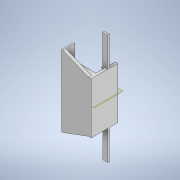
# Autodesk Inventor part: gira
Saved by Autodesk Inventor 2020 (Build 240168000, 168)
## iProperties
Created: 2022-10-31
Part Number: gira
Material: Generic
Document SubType Name: Modeling
Designer: super
Density: 1 g/cm^3
Appearance: Default
Author: super
Autodesk Inventor part; units mm, degrees
ref_plane "YZ Plane" through (0, 0, 0) normal (1, 0, 0) x (0, 1, 0)
ref_plane "XZ Plane" through (0, 0, 0) normal (0, 1, 0) x (-1, 0, 0)
ref_plane "XY Plane" through (0, 0, 0) normal (0, 0, 1) x (1, 0, 0)
ref_plane "Work Plane1" through (-84.5679, -177.7614, 10.4079) normal (0.999999, 0.0014131, 0) x (0.0014131, -0.999999, 0)
sketch "Sketch1" plane through (-84.5679, -177.7614, 10.4079) normal (0.999999, 0.0014131, 0) x (0.0014131, -0.999999, 0)
  line L0 (9.6295, -13.989) -> (-230.3705, -13.989)
  line L1 (-230.3705, -13.989) -> (-230.3705, 16.011)
  line L2 (-230.3705, 16.011) -> (9.6295, 16.011)
  line L3 (9.6295, 16.011) -> (9.6295, -13.989)
  point P0 (-177.6417, 10.4079)
  dimension "d40" = 240
  dimension "d41" = 30
  constraints: 8 end point, 2 parallel, 1 horizontal, 1 perpendicular
  measures "d40" distance of L0.start L0.end
  measures "d41" distance of L2.end L0.start
extrude "Extrusion1" add sketch "Sketch1" along normal blind 5
ref_plane "Work Plane2" through (-84.7238, -67.391, 24.3968) normal (-0.0014131, 0.999999, 0) x (0.999999, 0.0014131, 0)
sketch "Sketch3" plane through (-84.5543, -187.3909, 24.3968) normal (0, 0, 1) x (0.999999, 0.0014131, 0)
  line L0 (0, 0) -> (5, 0)
  line L1 (5, 0) -> (91.2544, 31.8306)
  line L2 (91.2544, 31.8306) -> (100.3623, 31.8306)
  line L3 (100.3623, 31.8306) -> (100.3623, 204.35)
  line L4 (100.3623, 204.35) -> (91.2544, 204.35)
  line L5 (5, 0) -> (5, 240) projected
  line L6 (91.2544, 204.35) -> (5, 240)
  line L7 (0, 0) -> (0, 240) projected
  line L8 (5, 240) -> (0, 240)
  line L9 (0, 240) -> (0, 0)
  point P0 (84.819, 187.2712)
  dimension "d42" = 172.5194
  dimension "d43" = 35.65
  constraints: 16 end point, 3 perpendicular, 2 parallel, 1 horizontal
  measures "d42" distance of L2.end L3.end
  measures "d43" vertical distance of L4.end L5.end
extrude "Extrusion2" add sketch "Sketch3" along normal blind 10
sketch "Sketch4" plane through (-84.5543, -187.3909, 24.3968) normal (0, 0, -1) x (-0.999999, -0.0014131, 0)
  line L0 (-100.3623, 204.35) -> (-91.2544, 204.35) projected
  line L1 (-91.2544, 31.8306) -> (-100.3623, 31.8306) projected
  line L2 (-100.3623, 204.35) -> (-91.2544, 204.35)
  line L3 (-91.2544, 204.35) -> (-91.2544, 31.8306)
  line L4 (-91.2544, 31.8306) -> (-100.3623, 31.8306)
  line L5 (-100.3623, 31.8306) -> (-100.3623, 204.35)
  point P0 (-84.819, 187.2712)
  point P1 (-100.3623, 31.8306)
  constraints: 8 end point, 2 parallel, 1 horizontal, 1 perpendicular
extrude "Extrusion3" add sketch "Sketch4" along normal blind 80
sketch "Sketch6" plane through (15.7629, -155.4186, -55.6032) normal (0.0014131, -0.999999, 0) x (0.999999, 0.0014131, 0)
  line L0 (0, 0) -> (0, 90) projected
  line L1 (0, 28.5548) -> (0, 34.1867)
  line L2 (0, 34.1867) -> (-17.3106, 34.1867)
  line L3 (-17.3106, 34.1867) -> (-17.3106, 28.5548)
  line L4 (-17.3106, 28.5548) -> (0, 28.5548)
  point P0 (-15.5433, 55.6032)
  constraints: 8 end point, 2 parallel, 2 point on line, 1 perpendicular
extrude "Extrusion5" add sketch "Sketch6" along normal blind 100
sketch "Sketch7" plane through (6.6551, -155.4314, -27.0484) normal (0, 0, -1) x (-0.999999, -0.0014131, 0)
  line L0 (8.2028, 0) -> (0, 14.7244)
  line L1 (0, 172.5194) -> (0, 0) projected
  line L2 (8.2028, 0) -> (0, 0) projected
  line L3 (0, 0) -> (8.2028, 0)
  constraints: 4 end point, 1 collinear, 1 point on line
extrude "Extrusion6" add sketch "Sketch7" against normal blind 10
ref_plane "Work Plane3" through (15.641, -69.1589, 34.3968) normal (-0.0014131, 0.999999, 0) x (0.999999, 0.0014131, 0)
mirror "Mirror1" about plane through (15.641, -69.1589, 34.3968) normal (-0.0014131, 0.999999, 0) of "Extrusion5", "Extrusion6"
ref_plane "Work Plane4" through (-84.7238, -67.391, -5.6032) normal (0.0014131, -0.999999, 0) x (0.999999, 0.0014131, 0)
sketch "Sketch10" plane through (-79.5679, -177.7543, 10.4079) normal (0.999999, 0.0014131, 0) x (0, 0, -1)
  point P0 (10.4079, 177.6417)
sketch "Sketch11" plane through (6.6551, -155.4314, -55.6032) normal (-0.999999, -0.0014131, 0) x (0, 0, 1)
  line L0 (80, 172.5194) -> (80, 0) projected
  line L1 (80, 172.5194) -> (64.9475, 172.5194)
  line L2 (64.9475, 172.5194) -> (64.9475, 165.7463)
  line L3 (64.9475, 165.7463) -> (80, 165.7463)
  line L4 (80, 165.7463) -> (80, 172.5194)
  point P0 (55.6032, 155.4407)
  point P1 (80, 165.7463)
  constraints: 8 end point, 2 parallel, 1 horizontal, 1 perpendicular
extrude "Extrusion7" add sketch "Sketch11" along normal blind 86.254
pattern_linear "Rectangular Pattern1" count 6 spacing 33 along (0.0014131, -0.999999, 0) of "Extrusion7"
sketch "Sketch14" plane through (-84.5679, -177.7614, 10.4079) normal (-0.999999, -0.0014131, 0) x (0, 0, 1)
  line L0 (23.989, 230.3705) -> (23.989, -9.6295) projected
  line L1 (23.989, -9.6295) -> (-16.011, -9.6295) projected
  point P0 (-10.4079, 177.6417)
  point P1 (-1.011, 10.3705)
  dimension "d38" = 25
  dimension "d39" = 20
  measures "d38" distance from line of L0 point (-1.011, 10.37)
  measures "d39" distance from line of L1 point (-1.011, 10.37)
hole "Hole2" at (-84.5825, -167.3909, 9.3968) direction (0.999999, 0.0014131, 0) diameter 10 depth 8 tip angle 118
body "Solid1"
